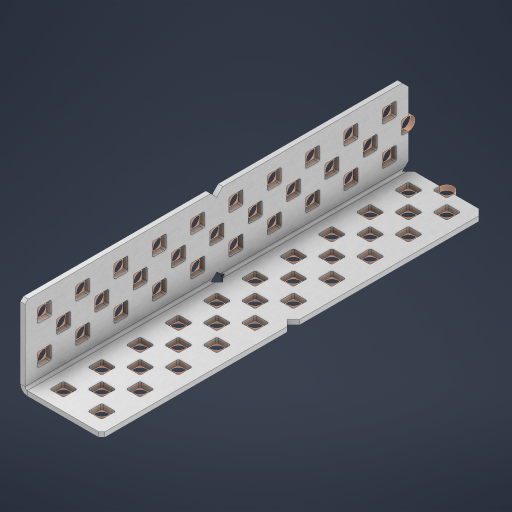
# Autodesk Inventor part: Alu C 1x2x1x35
Saved by Autodesk Inventor 2023 (Build 270158000, 158)
## iProperties
Created: 2022-07-28
Part Number: Alu C 1x2x1x35
Material: Generic
Document SubType Name: Sheet Metal
Designer: ylu12
Density: 1 g/cm^3
Sheet Metal Rule: Default
Appearance: Alu
Author: ylu12
Autodesk Inventor part; units mm, degrees
ref_plane "YZ Plane" through (0, 0, 0) normal (1, 0, 0) x (0, 1, 0)
ref_plane "XZ Plane" through (0, 0, 0) normal (0, 1, 0) x (-1, 0, 0)
sketch "Sketch1" plane through (0, 0, 0) normal (0, 1, 0) x (-1, 0, 0)
  line L0 (-12.7, 0) -> (12.7, 0)
  line L1 (12.7, 0) -> (12.7, -127)
  line L2 (12.7, -127) -> (-12.7, -127)
  line L3 (-12.7, -127) -> (-12.7, 0)
  line L4 (12.7, 0) -> (-12.7, -127) construction
  point P0 (0, 0)
  point P1 (0, 0)
  dimension "d0" = 25.4
  dimension "d1" = 127
  measures "d0" distance of L1.end L2.end
  measures "d1" distance of L0.end L1.end
extrude "Plate1" add sketch "Sketch1" along normal blind 1.5875
sketch "Sketch2" plane through (-12.7, 1.5875, 0) normal (-1, 0, 0) x (0, -1, 0)
  line L0 (0, -127) -> (0, 0)
  line L1 (0, 0) -> (-25.4, 0)
  line L2 (-25.4, 0) -> (-25.4, -127)
  line L3 (-25.4, -127) -> (0, -127)
  constraints: 6 end point, 1 horizontal, 1 perpendicular, 1 vertical
edge flange "Flanges" height 25.4 angle 90 thickness 1.5875 bend radius 0.7937 thickness toward (-1, 0, 0) relief tear relief width 1.5875 relief depth 0.7937 edges at (-12.7, 1.5875, -63.5) wall of the first edge with corners at (-12.7, 1.5875, -127) (-12.7, 1.5875, 0) (-12.7, 26.9875, 0) (-12.7, 26.9875, -127)
bend "Bend1"
corner "Corner1"
sketch "Sketch8" plane through (0, 0, 0) normal (0, -1, 0) x (1, 0, 0)
  line L0 (12.7, 0) -> (-11.9062, 0) construction
  line L1 (8.1534, -4.0386) -> (4.5466, -4.0386)
  line L2 (4.0386, -4.5466) -> (4.0386, -8.1534)
  line L3 (4.5466, -8.6614) -> (8.1534, -8.6614)
  line L4 (8.6614, -8.1534) -> (8.6614, -4.5466)
  arc A0 (8.6614, -4.5466) -> (8.1534, -4.0386) centre (8.1534, -4.5466) ccw
  arc A1 (8.1534, -8.6614) -> (8.6614, -8.1534) centre (8.1534, -8.1534) ccw
  arc A2 (4.0386, -8.1534) -> (4.5466, -8.6614) centre (4.5466, -8.1534) ccw
  arc A3 (4.5466, -4.0386) -> (4.0386, -4.5466) centre (4.5466, -4.5466) ccw
  line L5 (8.1534, -4.5466) -> (4.5466, -8.1534) construction
  line L6 (12.7, -127) -> (12.7, 0) construction
  point P0 (0, 0)
  point P1 (4.0386, -8.6614)
  point P2 (8.6614, -8.6614)
  point P3 (6.35, -6.35)
  dimension "d49" = 4.6228
  dimension "d50" = 0.508
  dimension "d52" = 6.35
  dimension "d123" = 6.35
  constraints: 10 end point, 8 point on circle, 8 tangent, 4 centre point, 4 point on line, 3 equal radius, 2 parallel, 2 perpendicular, 1 horizontal, 1 midpoint
  measures "d49" distance of point (8.661, -8.661) point (4.039, -8.661)
  measures "d50" radius of A0
  measures "d52" distance from line of L0 point (6.35, -6.35)
  measures "d123" distance from line of L6 point (6.35, -6.35)
extrude "Body Stamp" cut sketch "Sketch8" against normal blind 1.5875
sketch "Sketch9" plane through (0, 0, 0) normal (0, -1, 0) x (1, 0, 0)
  arc A0 (8.6614, -4.5466) -> (8.1534, -4.0386) centre (8.1534, -4.5466) ccw construction
  arc A1 (4.0386, -8.1534) -> (4.5466, -8.6614) centre (4.5466, -8.1534) ccw construction
  line L0 (8.1534, -4.5466) -> (4.5466, -8.1534) construction
  circle A2 centre (6.35, -6.35) radius 2.1844
  point P0 (0, 0)
  dimension "d55" = 4.3688
  constraints: 2 end point, 1 centre point, 1 midpoint
  measures "d55" diameter of A2
surface extrude "Body Circle" sketch "Sketch9" against normal up to surface (1.5875 mm away) shown yes curves A2
pattern_sketch "Body Pattern" of "Body Stamp", "Body Circle" from (6.35, 0, -6.35) copies at (6.35, 0, -19.05) at (6.35, 0, -31.75) at (6.35, 0, -44.45) at (-6.35, 0, -6.35) at (-6.35, 0, -19.05) at (-6.35, 0, -31.75) at (-6.35, 0, -44.45) at (6.35, 0, -57.15) at (-6.35, 0, -57.15) at (6.35, 0, -69.85) at (-6.35, 0, -69.85) at (6.35, 0, -82.55) at (-6.35, 0, -82.55) at (6.35, 0, -95.25) at (-6.35, 0, -95.25) at (6.35, 0, -107.95) at (-6.35, 0, -107.95) at (6.35, 0, -120.65) at (-6.35, 0, -120.65)
sketch "Sketch15" plane through (0, 0, 0) normal (0, -1, 0) x (1, 0, 0)
  line L0 (12.7, 0) -> (-11.9062, 0) construction
  line L1 (1.8034, -10.3886) -> (-1.8034, -10.3886)
  line L2 (-2.3114, -10.8966) -> (-2.3114, -14.5034)
  line L3 (-1.8034, -15.0114) -> (1.8034, -15.0114)
  line L4 (2.3114, -14.5034) -> (2.3114, -10.8966)
  arc A0 (2.3114, -10.8966) -> (1.8034, -10.3886) centre (1.8034, -10.8966) ccw
  arc A1 (1.8034, -15.0114) -> (2.3114, -14.5034) centre (1.8034, -14.5034) ccw
  arc A2 (-1.8034, -10.3886) -> (-2.3114, -10.8966) centre (-1.8034, -10.8966) ccw
  arc A3 (-2.3114, -14.5034) -> (-1.8034, -15.0114) centre (-1.8034, -14.5034) ccw
  line L5 (1.8034, -10.8966) -> (-1.8034, -14.5034) construction
  line L6 (12.7, 0) -> (12.7, -444.5) construction
  line L7 (0, 0) -> (0, -12.7) construction
  point P0 (10.3187, 0)
  point P1 (-2.3114, -15.0114)
  point P2 (2.3114, -15.0114)
  dimension "d106" = 4.6228
  dimension "d107" = 0.508
  dimension "d108" = 12.7
  constraints: 12 end point, 8 point on circle, 8 tangent, 4 centre point, 4 point on line, 3 equal radius, 2 parallel, 2 perpendicular, 1 horizontal, 1 midpoint, 1 vertical
  measures "d106" distance of point (2.311, -15.011) point (-2.311, -15.011)
  measures "d107" radius of A0
  measures "d108" distance from line of L0 L7.end
extrude "Center Stamp" cut sketch "Sketch15" against normal blind 1.5875
sketch "Sketch16" plane through (0, 0, 0) normal (0, -1, 0) x (1, 0, 0)
  circle A0 centre (0, -12.7) radius 2.1844
  line L0 (12.7, 0) -> (12.7, -444.5) construction
  arc A1 (-1.8034, -10.3886) -> (-2.3114, -10.8966) centre (-1.8034, -10.8966) ccw construction
  arc A2 (1.8034, -15.0114) -> (2.3114, -14.5034) centre (1.8034, -14.5034) ccw construction
  line L1 (-1.8034, -10.8966) -> (1.8034, -14.5034) construction
  point P0 (0, 0)
  point P1 (10.3187, 0)
  dimension "d112" = 4.3688
  constraints: 2 end point, 1 centre point, 1 coincident, 1 midpoint
  measures "d112" diameter of A0
surface extrude "Center Circle" sketch "Sketch16" against normal up to surface (1.5875 mm away) shown yes curves A0
pattern_linear "Center Pattern" count 10 spacing 12.7 along (0, 0, -1) of "Center Circle", "Center Stamp"
sketch "Arc Length" plane through (11.1125, 2.3813, 0) normal (0, 0, 1) x (1, 0, 0)
  line L0 (-25.4, 0) -> (-23.8125, 0) projected
  arc A0 (-25.4, 0) -> (-23.0187, -2.3813) centre (-23.0187, 0) ccw projected
  line L1 (-23.0187, -0.7938) -> (-23.0187, -2.3813) projected
  arc A1 (-23.8125, 0) -> (-23.0187, -0.7938) centre (-23.0187, 0) ccw projected
  point P0 (-11.1125, -2.3813)
  dimension "d126" = 1.2468
  dimension "d127" = 3.7405
sketch "Sketch13" plane through (-14.2875, 14.2875, 317.5) normal (1, 0, 0) x (0, 0, -1)
  line L0 (378.968, 12.7) -> (381, 10.668)
  line L1 (381, 10.668) -> (383.032, 12.7)
  line L2 (378.968, 12.7) -> (383.032, 12.7)
  line L3 (381, -10.8903) -> (378.7372, -13.1531)
  line L4 (378.7372, -13.1531) -> (381, -15.4159)
  line L5 (381, -15.4159) -> (383.2628, -13.1531)
  line L6 (383.2628, -13.1531) -> (381, -10.8903)
  line L7 (381, -10.8903) -> (381, -15.4159) construction
  line L8 (381, 10.668) -> (381, -10.8903) construction
  line L9 (444.5, 12.7) -> (317.5, 12.7) projected
  line L10 (444.5, -11.9062) -> (317.5, -11.9062) construction
  line L11 (317.5, 12.7) -> (317.5, -11.9062) construction
  point P0 (317.5, -14.2875)
  dimension "d86" = 4.5256
  dimension "d128" = 2.032
  dimension "d129" = 1.016
  dimension "d130" = 63.5
  constraints: 19 end point, 6 perpendicular, 2 vertical, 1 collinear
  measures "d86" distance of L3.start L4.end
  measures "d128" distance from line of L2 L0.end
  measures "d129" distance from line of L3.start L10
  measures "d130" distance between parallel lines of L11 L8
cut across bends "Notch" sketch "Sketch13" k factor 0.44
pattern_linear "Notch Pattern" count 2 spacing 63.5 along (0, 0, -1) of "Notch"
ref_plane "Diagonal Plane" through (-12.7, 1.5875, 0) normal (-0.7071068, 0.7071068, 0) x (0, 0, 1)
mirror "Everything Mirrored" about plane through (-12.7, 1.5875, 0) normal (-0.7071068, 0.7071068, 0) of "Body Stamp", "Body Circle", "Body Pattern", "Center Stamp", "Center Circle", "Center Pattern", "Notch", "Notch Pattern"
chamfer "End Chamfer" distance 1.016 angle 45 2 edges at (-13.4937, 26.9875, 0) (12.7, 0.7937, 0)
sketch "Body Pattern Sketch" plane through (0, 0, 0) normal (0, -1, 0) x (1, 0, 0)
  line L0 (12.7, 0) -> (-11.9062, 0) construction
  line L1 (12.7, 0) -> (12.7, -444.5) construction
  point P0 (0, 0)
  point P1 (6.35, -6.35)
  point P2 (6.35, -19.05)
  point P3 (6.35, -31.75)
  point P4 (6.35, -44.45)
  point P5 (-6.35, -6.35)
  point P6 (-6.35, -19.05)
  point P7 (-6.35, -31.75)
  point P8 (-6.35, -44.45)
  point P9 (6.35, -57.15)
  point P10 (-6.35, -57.15)
  point P11 (6.35, -69.85)
  point P12 (-6.35, -69.85)
  point P13 (6.35, -82.55)
  point P14 (-6.35, -82.55)
  point P15 (6.35, -95.25)
  point P16 (-6.35, -95.25)
  point P17 (6.35, -107.95)
  point P18 (-6.35, -107.95)
  point P19 (6.35, -120.65)
  point P20 (-6.35, -120.65)
  dimension "d62" = 12.7
  dimension "d65" = 12.7
  dimension "d99" = 6.35
  dimension "d125" = 6.35
  constraints: 1 horizontal, 1 vertical, 19 other
  measures "d99" distance from line of L0 point (6.35, -6.35)
  measures "d125" horizontal distance of point (0, 0) point (6.35, -6.35)
equation "\"d1\" = 12.7 * Length"
equation "\"d53\" = Thickness"
equation "\"d89\" = Thickness"
equation "\"JacobiRadiusSize\" = BendRadius"
equation "\"d2\" = Thickness"
equation "\"d3\" = BendReliefWidth"
equation "\"d4\" = BendReliefDepth"
equation "\"d5\" = MinimumRemnant"
equation "\"d6\" = TransitionRadius"
equation "\"d10\" = CornerReliefSize"
equation "\"d11\" = GapSize"
equation "\"d12\" = JacobiRadiusSize"
equation "\"BendRadius\" = Thickness"
equation "\"BendReliefWidth\" = Thickness"
equation "\"BendReliefDepth\" = 0.5 * Thickness"
equation "\"CornerReliefSize\" = 4 * Thickness"
equation "\"MinimumRemnant\" = 2 * Thickness"
equation "\"TransitionRadius\" = BendRadius"
equation "\"GapSize\" = Thickness"
equation "\"Length\" = 10"
equation "\"Thickness\" = 1.5875"
body "Solid1"
body "Srf91"
body "Srf92"
body "Srf786"
body "Srf856"
body "Srf857"
body "Srf858"
body "Srf859"
body "Srf860"
body "Srf861"
body "Srf889"
body "Srf890"
body "Srf891"
body "Srf1275"
body "Srf1276"
body "Srf1278"
body "Srf1279"
body "Srf1280"
body "Srf1281"
body "Srf1282"
body "Srf1283"
body "Srf1277"
body "Srf1285"
body "Srf1286"
body "Srf1287"
body "Srf1383"
body "Srf1384"
body "Srf1385"
body "Srf1386"
body "Srf1387"
body "Srf1388"
body "Srf1389"
body "Srf1390"
body "Srf1391"
body "Srf1392"
body "Srf1393"
body "Srf1394"
body "Srf1445"
body "Srf1446"
body "Srf1447"
body "Srf1448"
body "Srf1449"
body "Srf1450"
body "Srf1475"
body "Srf1476"
body "Srf1477"
body "Srf1478"
body "Srf1479"
body "Srf1480"
body "Srf1481"
body "Srf1482"
body "Srf1483"
body "Srf1484"
body "Srf1485"
body "Srf1486"
body "Srf1537"
body "Srf1538"
body "Srf1539"
body "Srf1540"
body "Srf1541"
body "Srf1542"
